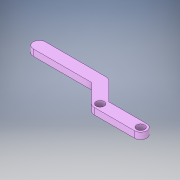
# Autodesk Inventor part: PINZA_DEDO
Saved by Autodesk Inventor 2019 (Build 230136000, 136)
## iProperties
Created: 2020-02-12
Part Number: PINZA_DEDO
Material: Genérico
Document SubType Name: Modeling
Designer: omar-
Density: 1 g/cm^3
Appearance: Valor por defecto
Author: omar-
Autodesk Inventor part; units mm, degrees
note: some values were not read from the file. Chosen so that the rebuilt part matches the saved one: sketch regions of "Extrusión1".
ref_plane "YZ Plane" through (0, 0, 0) normal (1, 0, 0) x (0, 1, 0)
ref_plane "XZ Plane" through (0, 0, 0) normal (0, 1, 0) x (-1, 0, 0)
ref_plane "XY Plane" through (0, 0, 0) normal (0, 0, 1) x (1, 0, 0)
sketch "Boceto1" plane through (0, 0, 0) normal (0, 1, 0) x (-1, 0, 0)
  circle A0 centre (0, 0) radius 2
  line L0 (0, 0) -> (20, 0) construction
  line L1 (0, -3) -> (20, -3)
  line L2 (20, 3) -> (0, 3)
  arc A1 (0, 3) -> (0, -3) centre (0, 0) ccw
  arc A2 (20, -3) -> (20, 3) centre (20, 0) ccw
  circle A3 centre (20, 0) radius 2
  line L3 (20, 0) -> (30, -10) construction
  line L4 (17.8787, -2.1213) -> (27.8787, -12.1213)
  line L5 (32.1213, -7.8787) -> (22.1213, 2.1213)
  arc A4 (22.1213, 2.1213) -> (17.8787, -2.1213) centre (20, 0) ccw
  arc A5 (27.8787, -12.1213) -> (32.1213, -7.8787) centre (30, -10) ccw
  line L6 (30, -10) -> (60, -10) construction
  line L7 (30, -13) -> (60, -13)
  line L8 (60, -7) -> (30, -7)
  arc A6 (30, -7) -> (30, -13) centre (30, -10) ccw
  arc A7 (60, -13) -> (60, -7) centre (60, -10) ccw
  point P0 (10, 0)
  point P1 (25, -5)
  point P2 (45, -10)
  dimension "d0" = 4
  dimension "d1" = 6
  dimension "d2" = 20
  dimension "d3" = 4
  dimension "d4" = 6
  dimension "d5" = 5
  dimension "d6" = 5
  dimension "d7" = 6
  dimension "d8" = 30
  constraints: 24 end point, 12 point on circle, 12 tangent, 8 centre point, 3 midpoint, 3 parallel, 2 coincident, 2 horizontal
  measures "d0" diameter of A0
  measures "d1" diameter of A2
  measures "d2" distance of L1.start L1.end
  measures "d3" diameter of A3
  measures "d4" diameter of A5
  measures "d5" horizontal distance of point (25, -5) L0.end
  measures "d6" horizontal distance of point (25, -5) L3.start
  measures "d7" diameter of A7
  measures "d8" distance of L7.start L7.end
extrude "Extrusión1" add sketch "Boceto1" along normal blind 3.18
